Autodesk Fusion 360 part; units mm, degrees
(part 3 of 3)
  measures "d247" diameter of A8
  measures "d248" diameter of A9
  measures "d249" diameter of A10
  measures "d250" diameter of A11
  measures "d251" diameter of A12
  measures "d252" diameter of A13
  measures "d253" diameter of A14
  measures "d254" diameter of A15
  measures "d255" diameter of A16
  measures "d256" diameter of A17
  measures "d257" diameter of A18
  measures "d258" diameter of A19
  measures "d259" diameter of A20
  measures "d260" diameter of A21
  measures "d261" diameter of A22
  measures "d262" diameter of A23
  measures "d263" diameter of A24
  measures "d281" distance of P2 L243.end
  measures "d282" distance of L243.end L244.end
  measures "d283" diameter of A25
  measures "d284" distance of L250.start L249.end
  measures "d285" distance of L250.end L250.start
  measures "d286" diameter of A26
  measures "d287" distance of L255.end L256.end
  measures "d288" distance of L255.start L255.end
  measures "d289" diameter of A30
  measures "d290" diameter of A27
  measures "d291" diameter of A28
  measures "d292" diameter of A29
  measures "d293" distance of L258 L262
  measures "d294" distance of L255 L261
  measures "d295" distance of L276.end L277.end
  measures "d296" distance of L275.end L276.end
  measures "d297" distance of L272.end L273.end
  measures "d298" distance of L271.end L272.end
  measures "d299" distance of L267.start L269.end
extrude "Extruir15" add sketch "Boceto15" along normal blind 4 contours L260 L261 L267 L269 L270 | L259 L260 L271 L272 L273 L274 | L261 L262 L263 L264 L265 L266 | L259 L262 L275 L276 L277 L278 | L151 L152 L153 L154 L157 L158 | L156 L157 L159 L160 L161 L162 | L155 L158 L163 L164 L165 L166 | L155 L156 L167 L168 L169 L170 | L171 L172 L173 L174 | L175 L176 L177 L178 | L179 L180 L181 L182 | L183 L184 L185 L186 | L187 L188 L189 L190 | L191 L192 L193 L194 | L195 L196 L197 L198 | L199 L200 L201 L202 | L203 L204 L205 L206 | L207 L208 L209 L210 | L211 L212 L213 L214 | L215 L216 L217 L218 | L227 L228 L229 L230 | L231 L232 L233 L234 | L235 L236 L237 L238 | L239 L240 L241 L242 | L243 L244 L245 L246 | L249 L250 L252 L254
sketch "Boceto17" plane through (0, 0, 5) normal (0, 0, 1) x (-1, 0, 0)
  circle A0 centre (12, -97) radius 1.5
  circle A1 centre (-162, -97) radius 1.5
  circle A2 centre (12, -3) radius 1.5
  circle A3 centre (-162, -42) radius 1.5
  circle A4 centre (8.65, -85.637) radius 1.6
  circle A5 centre (8.65, -71.337) radius 1.6
  circle A6 centre (-97.75, -72.95) radius 1
  circle A7 centre (-145.75, -75.7793) radius 0.75
  circle A8 centre (-156.15, -6.35) radius 1
  circle A9 centre (-65.25, -19.25) radius 1.5
  circle A10 centre (-24.75, -19.25) radius 1.5
  circle A11 centre (-57.75, -19.25) radius 1.5
  circle A12 centre (-134.75, -64.25) radius 1.5
  circle A13 centre (-155.65, -50.85) radius 1
  circle A14 centre (-104.75, -91.2793) radius 0.75
  circle A15 centre (-77.75, -72.95) radius 1
  circle A16 centre (-16.9746, -57.735) radius 1.4
  circle A17 centre (4.6254, -28.735) radius 1.4
  circle A18 centre (4.6254, -57.735) radius 1.25
  circle A19 centre (-97.75, -89.75) radius 1
  circle A20 centre (-145.75, -91.2793) radius 0.75
  circle A21 centre (-141.85, -6.35) radius 1
  circle A22 centre (-65.25, -64.25) radius 1.5
  circle A23 centre (-24.75, -64.25) radius 1.5
  circle A24 centre (-57.75, -64.25) radius 1.5
  circle A25 centre (-134.75, -19.25) radius 1.5
  circle A26 centre (-155.75, -65.15) radius 1
  circle A27 centre (-104.75, -75.7793) radius 0.75
  circle A28 centre (-77.75, -89.75) radius 1
  circle A29 centre (-16.9746, -28.735) radius 1.4
  line L0 (-165, 0) -> (-165, -77.5293)
extrude "Extruir24" cut sketch "Boceto17" against normal blind 90 contours A0 | A1 | A2 | A3
sketch "Boceto16" plane through (0, 0, 5) normal (0, 0, 1) x (-1, 0, 0)
  line L0 (-157.5, -63) -> (-159, -63)
  line L1 (-165, -77.5293) -> (-147, -77.5293)
  line L2 (-147, -77.5293) -> (-147, -77.0293)
  line L3 (-144.5, -74.5293) -> (-106, -74.5293)
  line L4 (-103.5, -77.0293) -> (-103.5, -90.0293)
  line L5 (-106, -92.5293) -> (-144.5, -92.5293)
  line L6 (-147, -89.5293) -> (-165, -89.5293)
  line L7 (-165, -89.5293) -> (-165, -100)
  line L8 (-165, -100) -> (15, -100)
  line L9 (15, -100) -> (15, 0)
  line L10 (10.5, -83.487) -> (10.5, -83.787)
  line L11 (6.8, -87.487) -> (-7.5, -87.487)
  line L12 (-7.5, -87.487) -> (-7.5, -69.487)
  line L13 (-7.5, -69.487) -> (6.8, -69.487)
  line L14 (10.5, -73.487) -> (12, -73.487)
  line L15 (15, 0) -> (-165, 0)
  line L16 (-144, -3) -> (-144, -4.5)
  line L17 (-140, -8.2) -> (-140, -22.5)
  line L18 (-140, -22.5) -> (-158, -22.5)
  line L19 (-158, -22.5) -> (-158, -8.2)
  line L20 (-154, -4.5) -> (-154, -3)
  line L21 (-159, -53) -> (-157.5, -53)
  line L22 (-157.5, -53) -> (-157.5, -52.7)
  line L23 (-153.8, -49) -> (-139.5, -49)
  line L24 (-139.5, -49) -> (-139.5, -67)
  line L25 (-139.5, -67) -> (-153.8, -67)
  line L26 (-60.5, -61.5) -> (-60.5, -22)
  line L27 (-55, -16.5) -> (-27.5, -16.5)
  line L28 (-22, -22) -> (-22, -61.5)
  line L29 (-27.5, -67) -> (-55, -67)
  line L30 (-100.5, -87) -> (-100.5, -75.7)
  line L31 (-95, -70.2) -> (-80.5, -70.2)
  line L32 (-75, -75.7) -> (-75, -87)
  line L33 (-80.5, -92.5) -> (-95, -92.5)
  line L34 (-72.5, -92.5) -> (-72.5, -69)
  line L35 (-72.5, -69) -> (-22, -69)
  line L36 (-22, -69) -> (-22, -92.5)
  line L37 (-22, -92.5) -> (-72.5, -92.5)
  line L38 (-19.3746, -53.685) -> (-19.3746, -32.785)
  line L39 (-13.3746, -24.785) -> (1.0254, -24.785)
  line L40 (7.0254, -32.785) -> (7.0254, -53.685)
  line L41 (1.0254, -61.685) -> (-13.3746, -61.685)
  line L42 (-137.5, -61.5) -> (-137.5, -22)
  line L43 (-132, -16.5) -> (-68, -16.5)
  line L44 (-62.5, -22) -> (-62.5, -61.5)
  line L45 (-68, -67) -> (-132, -67)
  line L46 (-132.793, -73.7793) -> (-132.793, -67.7793)
  line L47 (-132.793, -67.7793) -> (-112.793, -67.7793)
  line L48 (-112.793, -67.7793) -> (-112.793, -73.7793)
  line L49 (-112.793, -73.7793) -> (-132.793, -73.7793)
  line L50 (163.4623, -50) -> (102.1469, -50)
  line L51 (102.1469, -50) -> (102.1469, -3.728)
  line L52 (102.1469, -3.728) -> (163.4623, -3.728)
  line L53 (163.4623, -3.728) -> (163.4623, -50)
  circle A0 centre (158.4623, -45) radius 1.5
  line L54 (163.4623, -40) -> (158.4623, -40)
  line L55 (153.4623, -50) -> (153.4623, -45)
  arc A1 (158.4623, -40) -> (153.4623, -45) centre (158.4623, -45) ccw
  line L56 (9, 0) -> (9, -3)
  line L57 (12, -6) -> (12, -6)
  arc A2 (15, -3.0005) -> (15, -2.9995) centre (12, -3) ccw
  arc A3 (9, -3) -> (12, -6) centre (12, -3) ccw
  line L58 (-162, -45) -> (-165, -45)
  line L59 (-165, -39) -> (-162, -39)
  arc A4 (-162, -45) -> (-162, -39) centre (-162, -42) ccw
  line L60 (-154.4341, -89.5293) -> (-154.4341, -77.5293)
  line L61 (-162, -94) -> (-160, -94)
  line L62 (-159, -100) -> (-159, -97)
  arc A5 (-159, -97) -> (-162, -94) centre (-162, -97) ccw
  line L63 (15, -94) -> (12, -94)
  line L64 (9, -100) -> (9, -97)
  arc A6 (12, -94) -> (9, -97) centre (12, -97) ccw
  line L65 (12, -97) -> (-162, -97)
  line L66 (-162, -97) -> (-162, -3)
  line L67 (-162, -3) -> (12, -3)
  line L68 (12, -3) -> (12, -97)
  line L69 (12, -73.487) -> (12, -83.487)
  line L70 (12, -83.487) -> (10.5, -83.487)
  line L71 (-159, -63) -> (-159, -53)
  line L72 (-154.3, -4.5) -> (-154, -4.5)
  line L73 (-154, -3) -> (-144, -3)
  line L74 (-165, -89.5293) -> (-165, -77.5293)
  circle A7 centre (12, -97) radius 1.5
  circle A8 centre (-162, -97) radius 1.5
  circle A9 centre (12, -3) radius 1.5
  circle A10 centre (-162, -42) radius 1.5
  circle A11 centre (8.65, -85.637) radius 1.6
  circle A12 centre (8.65, -71.337) radius 1.6
  circle A13 centre (-97.75, -72.95) radius 1
  circle A14 centre (-145.75, -75.7793) radius 0.75
  circle A15 centre (-156.15, -6.35) radius 1
  circle A16 centre (-65.25, -19.25) radius 1.5
  circle A17 centre (-24.75, -19.25) radius 1.5
  circle A18 centre (-57.75, -19.25) radius 1.5
  circle A19 centre (-134.75, -64.25) radius 1.5
  circle A20 centre (-155.65, -50.85) radius 1
  circle A21 centre (-104.75, -91.2793) radius 0.75
  circle A22 centre (-77.75, -72.95) radius 1
  circle A23 centre (-16.9746, -57.735) radius 1.4
  circle A24 centre (4.6254, -28.735) radius 1.4
  circle A25 centre (4.6254, -57.735) radius 1.25
  circle A26 centre (-97.75, -89.75) radius 1
  circle A27 centre (-145.75, -91.2793) radius 0.75
  circle A28 centre (-141.85, -6.35) radius 1
  circle A29 centre (-65.25, -64.25) radius 1.5
  circle A30 centre (-24.75, -64.25) radius 1.5
  circle A31 centre (-57.75, -64.25) radius 1.5
  circle A32 centre (-134.75, -19.25) radius 1.5
  circle A33 centre (-155.75, -65.15) radius 1
  circle A34 centre (-104.75, -75.7793) radius 0.75
  circle A35 centre (-77.75, -89.75) radius 1
  circle A36 centre (-16.9746, -28.735) radius 1.4
  line L75 (-147, -77.0293) -> (-144.5, -77.0293)
  line L76 (-144.5, -77.0293) -> (-144.5, -74.5293)
  line L77 (-106, -74.5293) -> (-106, -77.0293)
  line L78 (-106, -77.0293) -> (-103.5, -77.0293)
  line L79 (-103.5, -90.0293) -> (-106, -90.0293)
  line L80 (-106, -90.0293) -> (-106, -92.5293)
  line L81 (-144.5, -92.5293) -> (-144.5, -90.0293)
  line L82 (-144.5, -90.0293) -> (-147, -90.0293)
  line L83 (-147, -90.0293) -> (-147, -89.5293)
  line L84 (-165, 0) -> (-165, -77.5293)
  line L85 (10.5, -83.787) -> (6.8, -83.787)
  line L86 (6.8, -83.787) -> (6.8, -87.487)
  line L87 (6.8, -69.487) -> (6.8, -73.187)
  line L88 (6.8, -73.187) -> (10.5, -73.187)
  line L89 (10.5, -73.187) -> (10.5, -73.487)
  line L90 (-137.5, -22) -> (-132, -22)
  line L91 (-132, -22) -> (-132, -16.5)
  line L92 (-68, -16.5) -> (-68, -22)
  line L93 (-68, -22) -> (-62.5, -22)
  line L94 (-62.5, -61.5) -> (-68, -61.5)
  line L95 (-68, -61.5) -> (-68, -67)
  line L96 (-132, -67) -> (-132, -61.5)
  line L97 (-132, -61.5) -> (-137.5, -61.5)
  line L98 (-19.3746, -32.785) -> (-13.3746, -32.785)
  line L99 (-13.3746, -32.785) -> (-13.3746, -24.785)
  line L100 (1.0254, -24.785) -> (1.0254, -32.785)
  line L101 (1.0254, -32.785) -> (7.0254, -32.785)
  line L102 (7.0254, -53.685) -> (1.0254, -53.685)
  line L103 (1.0254, -53.685) -> (1.0254, -61.685)
  line L104 (-13.3746, -61.685) -> (-13.3746, -53.685)
  line L105 (-13.3746, -53.685) -> (-19.3746, -53.685)
  line L106 (-144, -4.5) -> (-143.7, -4.5)
  line L107 (-143.7, -4.5) -> (-143.7, -8.2)
  line L108 (-143.7, -8.2) -> (-140, -8.2)
  line L109 (-158, -8.2) -> (-154.3, -8.2)
  line L110 (-154.3, -8.2) -> (-154.3, -4.5)
  line L111 (-100.5, -75.7) -> (-95, -75.7)
  line L112 (-95, -75.7) -> (-95, -70.2)
  line L113 (-80.5, -70.2) -> (-80.5, -75.7)
  line L114 (-80.5, -75.7) -> (-75, -75.7)
  line L115 (-75, -87) -> (-80.5, -87)
  line L116 (-80.5, -87) -> (-80.5, -92.5)
  line L117 (-95, -92.5) -> (-95, -87)
  line L118 (-95, -87) -> (-100.5, -87)
  line L119 (-60.5, -22) -> (-55, -22)
  line L120 (-55, -22) -> (-55, -16.5)
  line L121 (-27.5, -16.5) -> (-27.5, -22)
  line L122 (-27.5, -22) -> (-22, -22)
  line L123 (-22, -61.5) -> (-27.5, -61.5)
  line L124 (-27.5, -61.5) -> (-27.5, -67)
  line L125 (-55, -67) -> (-55, -61.5)
  line L126 (-55, -61.5) -> (-60.5, -61.5)
  line L127 (-157.5, -52.7) -> (-153.8, -52.7)
  line L128 (-153.8, -52.7) -> (-153.8, -49)
  line L129 (-153.8, -67) -> (-153.8, -63.3)
  line L130 (-153.8, -63.3) -> (-157.5, -63.3)
  line L131 (-157.5, -63.3) -> (-157.5, -63)
  dimension "d302" = 5
  dimension "d303" = 5
  dimension "d304" = 10
  dimension "d305" = 3
  dimension "d306" = 3
  dimension "d307" = 3
  constraint horizontal L50
  constraint vertical L51
  constraint horizontal L52
  constraint vertical L53
  constraint concentric A0 A1
  constraint coincident L53 L54.start
  constraint perpendicular L53 L54
  constraint coincident L50 L55.start
  constraint perpendicular L50 L55
  constraint tangent L55 A1
  constraint tangent L54 A1
  constraint tangent L15 A2
  constraint coincident L15 L56.start
  constraint perpendicular L15 L56
  constraint tangent L57 A2
  constraint tangent L56 A2
  constraint coincident L56.end A2
  constraint concentric A2 A3
  constraint tangent L59 A4
  constraint tangent L58 A4
  constraint coincident L6 L60.start
  constraint coincident L1 L60.end
  constraint perpendicular L1 L60
  constraint tangent L8 A5
  constraint coincident L61.start A5
  constraint horizontal L61
  constraint coincident L8 L62.start
  constraint perpendicular L8 L62
  constraint tangent L62 A5
  constraint coincident L61 A5.end
  constraint tangent L9 A6
  constraint coincident L9 L63.start
  constraint perpendicular L9 L63
  constraint coincident L8 L64.start
  constraint perpendicular L8 L64
  constraint tangent L64 A6
  constraint tangent L63 A6
  constraint horizontal L65
  constraint vertical L66
  constraint horizontal L67
  constraint vertical L68
  constraint coincident L68 L57.start
  measures "d302" distance of L50 A0.centre
  measures "d303" distance of L53 A0.centre
  measures "d304" diameter of A1
  measures "d305" diameter of A0
  measures "d306" distance of L15 L67
  measures "d307" distance of L8 L65
extrude "Extruir23" add sketch "Boceto16" along normal blind 50 contours L1 L6 L66 L74 | L1 L58 L66 L84 | L6 L7 L8 L62 L65 L66 A8 | A4 L66 A10 | L58 L59 L66 A10 L84 | A5 L65 L66 A8 | L15 L56 L59 L66 L67 L73 L84 | L8 L62 L64 L65 | L8 L9 L63 L64 L65 L68 A7 | A6 L65 L68 A7 | L15 L56 A2 | L9 A2 L63 L68 L69 | L9 L15 A2 | A2 L67 L68 A9 | A2 A3 L67 L68 A9
extrude "Extruir25" add 1 faces at (163, 85.5293, 5) along direction (0, 0, -1) blind 4
sketch "Boceto18" plane through (165, 0, 0) normal (1, 0, 0) x (0, 1, 0)
  line L0 (100, 0) -> (100, 55)
  line L1 (100, 55) -> (0, 55)
  line L2 (0, 55) -> (0, 0)
  line L3 (0, 0) -> (100, 0)
  line L4 (49, 1) -> (52.7, 1) construction
  line L5 (52.7, 1) -> (53, 1) construction
  line L6 (53, 1) -> (63, 1) construction
  line L7 (63, 1) -> (63.3, 1) construction
  line L8 (63.3, 1) -> (67, 1) construction
  line L9 (67, 1) -> (49, 1) construction
  line L10 (53.45, 5) -> (62.55, 5) construction
  line L11 (62.55, 5) -> (62.55, 2) construction
  line L12 (62.55, 2) -> (53.45, 2) construction
  line L13 (53.45, 2) -> (53.45, 5) construction
  line L14 (58, 1) -> (58, 2) construction
  line L15 (54.95, 2) -> (61.05, 2) construction
  arc A0 (61.05, 2) -> (61.05, 5) centre (61.05, 3.5) ccw construction
  line L16 (61.05, 5) -> (54.95, 5) construction
  arc A1 (54.95, 5) -> (54.95, 2) centre (54.95, 3.5) ccw construction
  line L17 (53.45, 3.5) -> (62.55, 3.5) construction
  arc A2 (61.05, -1) -> (61.05, 8) centre (61.05, 3.5) ccw
  line L18 (61.05, 8) -> (54.95, 8)
  arc A3 (54.95, 8) -> (54.95, -1) centre (54.95, 3.5) ccw
  line L19 (54.95, -1) -> (61.05, -1)
  line L20 (50.45, 3.5) -> (50.45, 0)
  line L21 (65.55, 3.5) -> (65.55, 0)
  point P0 (49, 1)
  dimension "d322" = 1
  dimension "d323" = 3
  dimension "d324" = 9.1
  dimension "d325" = 3
  constraint horizontal L10
  constraint vertical L11
  constraint horizontal L12
  constraint vertical L13
  constraint midpoint L6 L14.start
  constraint midpoint L12 L14.end
  constraint vertical L14
  constraint tangent L15 A0
  constraint tangent A0 L16
  constraint parallel L15 L16
  constraint tangent L16 A1
  constraint tangent L15 A1
  constraint midpoint A1 L17.start
  constraint midpoint A0 L17.end
  constraint midpoint L11 L17.end
  constraint perpendicular L11 L17
  constraint midpoint L13 L17.start
  constraint midpoint A3 L20.start
  constraint coincident L3 L20.end
  constraint tangent A3 L20
  constraint perpendicular L3 L20
  constraint midpoint A2 L21.start
  constraint coincident L3 L21.end
  constraint tangent A2 L21
  constraint perpendicular L3 L21
  measures "d322" distance of L9 L12
  measures "d323" distance of L10.end L11.end
  measures "d324" distance of L10.start L10.end
extrude "Extruir26" cut sketch "Boceto18" against normal blind 6 contours L3 A2 L21 | L3 A2 L18 A3 | L3 A3 L20
sketch "Boceto19" plane through (0, 0, 0) normal (0, -1, 0) x (1, 0, 0)
  line L0 (-15, 0) -> (165, 0)
  line L1 (165, 0) -> (165, 55)
  line L2 (165, 55) -> (-15, 55)
  line L3 (-15, 55) -> (-15, 0)
  line L4 (152.0391, 4.1783) -> (145.9609, 4.1783) construction
  line L5 (140.8268, 0.1675) -> (144.0809, 1) construction
  line L6 (144.45, 1.1675) -> (144.45, 4.1675) construction
  line L7 (145.9609, 1.1566) -> (152.0391, 1.1566) construction
  line L8 (153.9217, 1) -> (157.1517, 0.1675) construction
  line L9 (144.45, 4.1675) -> (153.55, 4.1675) construction
  line L10 (152.0391, 7.1783) -> (145.9608, 7.1783)
  arc A0 (145.9609, 4.1783) -> (145.9609, 1.1566) centre (145.9609, 2.6675) ccw construction
  line L11 (141.45, 2.6675) -> (141.45, -2.9323)
  line L12 (148.9999, 1) -> (153.9217, 1) construction
  line L13 (144.0809, 1) -> (149.0001, 1) construction
  line L14 (144.45, 2.6675) -> (153.55, 2.6675) construction
  arc A1 (152.0392, -1.8434) -> (152.0391, 7.1783) centre (152.0391, 2.6675) ccw
  line L15 (149.0001, 1) -> (148.9999, 1) construction
  line L16 (153.55, 4.1675) -> (153.55, 1.1675) construction
  line L17 (157.1517, 0.1675) -> (140.8268, 0.1675) construction
  arc A2 (152.0391, 1.1566) -> (152.0391, 4.1783) centre (152.0391, 2.6675) ccw construction
  arc A3 (145.9608, 7.1783) -> (145.9608, -1.8434) centre (145.9609, 2.6675) ccw
  line L18 (153.55, 1.1675) -> (144.45, 1.1675) construction
  line L19 (156.55, 2.6675) -> (156.5501, -3.4458)
  line L20 (145.9608, -1.8434) -> (152.0392, -1.8434)
  line L21 (149, 1) -> (149, 1.1675) construction
  line L22 (154.3, 1) -> (158, 1) construction
  line L23 (158, 1) -> (140, 1) construction
  line L24 (140, 1) -> (143.7, 1) construction
  line L25 (143.7, 1) -> (144, 1) construction
  line L26 (144, 1) -> (154, 1) construction
  line L27 (154, 1) -> (154.3, 1) construction
  point P0 (61.5347, -18.624)
  point P1 (149, 1)
  dimension "d328" = 3
  dimension "d329" = 1
  dimension "d330" = 3
  dimension "d331" = 9.1
  constraint horizontal L9
  constraint vertical L16
  constraint horizontal L18
  constraint vertical L6
  constraint midpoint P1 L15
  constraint midpoint L21.end L18
  constraint vertical L21
  constraint tangent L7 A2
  constraint tangent L4 A2
  constraint parallel L4 L7
  constraint tangent L4 A0
  constraint tangent L7 A0
  constraint midpoint L14.start A0
  constraint midpoint L14.end A2
  constraint midpoint L14.end L16
  constraint perpendicular L14 L16
  constraint midpoint L14.start L6
  constraint midpoint L11.start A3
  constraint tangent L11 A3
  constraint midpoint L19.start A1
  constraint tangent A1 L19
  constraint midpoint L26 P1
  constraint coincident P1 L21.start
  measures "d329" distance of L17 L18
  measures "d330" distance of L16.end L9.end
  measures "d331" distance of L6.end L9.end
extrude "Extruir27" cut sketch "Boceto19" against normal blind 3 contours L0 L11 A3 | L0 L10 A1 A3 | L0 A1 L19
sketch "Boceto20" plane through (-15, 0, 0) normal (-1, 0, 0) x (0, -1, 0)
  line L0 (-100, 0) -> (0, 0)
  line L1 (0, 0) -> (0, 55)
  line L2 (0, 55) -> (-2.9995, 55)
  line L3 (-2.9995, 55) -> (-2.9995, 5)
  line L4 (-2.9995, 5) -> (-3.0005, 5)
  line L5 (-3.0005, 55) -> (-100, 55)
  line L6 (-100, 55) -> (-100, 0)
  line L7 (-75.437, 5) -> (-81.537, 5) construction
  line L8 (-87.487, 1) -> (-83.787, 1) construction
  line L9 (-83.037, 2) -> (-83.037, 5) construction
  line L10 (-81.537, 2) -> (-75.437, 2) construction
  line L11 (-73.187, 1) -> (-69.487, 1) construction
  line L12 (-83.037, 5) -> (-73.937, 5) construction
  line L13 (-75.437, 8) -> (-81.537, 8)
  arc A0 (-81.537, 5) -> (-81.537, 2) centre (-81.537, 3.5) ccw construction
  line L14 (-86.037, 3.5) -> (-86.037, 0)
  line L15 (-73.487, 1) -> (-73.187, 1) construction
  line L16 (-83.787, 1) -> (-83.487, 1) construction
  line L17 (-83.037, 3.5) -> (-73.937, 3.5) construction
  arc A1 (-75.437, -1) -> (-75.437, 8) centre (-75.437, 3.5) ccw
  line L18 (-83.487, 1) -> (-73.487, 1) construction
  line L19 (-73.937, 5) -> (-73.937, 2) construction
  line L20 (-69.487, 1) -> (-87.487, 1) construction
  arc A2 (-75.437, 2) -> (-75.437, 5) centre (-75.437, 3.5) ccw construction
  arc A3 (-81.537, 8) -> (-81.537, -1) centre (-81.537, 3.5) ccw
  line L21 (-73.937, 2) -> (-83.037, 2) construction
  line L22 (-70.937, 3.5) -> (-70.937, 0)
  line L23 (-81.537, -1) -> (-75.437, -1)
  line L24 (-78.487, 1) -> (-78.487, 2) construction
  line L25 (-87.487, 1) -> (-83.787, 1) construction
  line L26 (-83.787, 1) -> (-83.487, 1) construction
  line L27 (-83.487, 1) -> (-73.487, 1) construction
  line L28 (-73.487, 1) -> (-73.187, 1) construction
  line L29 (-73.187, 1) -> (-69.487, 1) construction
  line L30 (-69.487, 1) -> (-87.487, 1) construction
  line L31 (-3.0005, 5) -> (-3.0005, 55)
  point P0 (49, 1)
  point P1 (-78.487, 1)
  dimension "d334" = 3
  dimension "d335" = 1
  dimension "d336" = 3
  dimension "d337" = 9.1
  constraint horizontal L12
  constraint vertical L19
  constraint horizontal L21
  constraint vertical L9
  constraint midpoint P1 L18
  constraint midpoint L24.end L21
  constraint vertical L24
  constraint tangent L10 A2
  constraint tangent L7 A2
  constraint parallel L7 L10
  constraint tangent L7 A0
  constraint tangent L10 A0
  constraint midpoint L17.start A0
  constraint midpoint L17.end A2
  constraint midpoint L17.end L19
  constraint perpendicular L17 L19
  constraint midpoint L17.start L9
  constraint midpoint L14.start A3
  constraint tangent L14 A3
  constraint midpoint L22.start A1
  constraint tangent A1 L22
  constraint midpoint L27 P1
  constraint coincident P1 L24.start
  measures "d335" distance of L20 L21
  measures "d336" distance of L19.end L12.end
  measures "d337" distance of L9.end L12.end
extrude "Extruir28" cut sketch "Boceto20" against normal blind 3 contours L0 L14 A3 | L0 L13 A1 A3 | L0 A1 L22
sketch "Boceto21" plane through (0, 0, 0) normal (0, -1, 0) x (1, 0, 0)
  line L0 (156.55, 2.6675) -> (156.5501, 0)
  line L1 (156.5501, 0) -> (165, 0)
  line L2 (165, 0) -> (165, 55)
  line L3 (165, 55) -> (-15, 55)
  line L4 (-15, 55) -> (-15, 0)
  line L5 (-15, 0) -> (141.45, 0)
  line L6 (141.45, 0) -> (141.45, 2.6675)
  arc A0 (145.9608, 7.1783) -> (141.45, 2.6675) centre (145.9609, 2.6675) ccw
  line L7 (145.9608, 7.1783) -> (152.0391, 7.1783)
  arc A1 (156.55, 2.6675) -> (152.0391, 7.1783) centre (152.0391, 2.6675) ccw
  circle A2 centre (70.8934, 40) radius 9.75
  circle A3 centre (129.1066, 40) radius 6.45
  line L8 (62.5, 5) -> (137.5, 5) construction
  line L9 (100, 5) -> (100, 40) construction
  line L10 (70.8934, 40) -> (129.1066, 40) construction
  point P0 (62.5, 5)
  point P1 (137.5, 5)
  dimension "d340" = 19.5
  dimension "d341" = 12.9
  dimension "d342" = 35
  constraint coincident P0 L8.start
  constraint coincident P1 L8.end
  constraint midpoint L8 L9.start
  constraint perpendicular L8 L9
  constraint coincident A2.centre L10.start
  constraint coincident A3.centre L10.end
  constraint horizontal L10
  constraint midpoint L9.end L10
  measures "d340" diameter of A2
  measures "d341" diameter of A3
  measures "d342" distance of L9.start L9.end
extrude "Extruir29" cut sketch "Boceto21" against normal blind 3 contours A2 | A3
sketch "Boceto22" plane through (0, 100, 0) normal (0, 1, 0) x (-1, 0, 0)
  line L0 (-165, 0) -> (15, 0)
  line L1 (15, 0) -> (15, 55)
  line L2 (15, 55) -> (-165, 55)
  line L3 (-165, 55) -> (-165, 0)
  line L4 (-72.5, 5) -> (-72.5, 6)
  line L5 (-72.5, 6) -> (-72.5, 33) construction
  line L6 (-22, 5) -> (-22, 34.9) construction
  circle A0 centre (-22, 37.1) radius 1.8
  circle A1 centre (-22, 17.9) radius 1.8
  line L7 (-22, 37.1) -> (-22, 17.9) construction
  line L8 (-22, 27.5) -> (15, 27.5) construction
  line L9 (-22, 27.5) -> (-79, 27.5) construction
  circle A2 centre (-72.5, 27.5) radius 2
  point P0 (-72.5, 5)
  point P1 (-22, 5)
  dimension "d345" = 3.6
  dimension "d346" = 3.6
  dimension "d347" = 19.2
  dimension "d350" = 4
  constraint coincident P0 L4.start
  constraint perpendicular L0 L4
  constraint perpendicular L0 L5
  constraint coincident P1 L6.start
  constraint perpendicular L0 L6
  constraint coincident L6 A0.centre
  constraint coincident L6 A1.centre
  constraint coincident A0.centre L7.start
  constraint coincident A1.centre L7.end
  constraint midpoint L7 L8.start
  constraint midpoint L1 L8.end
  constraint horizontal L8
  constraint perpendicular L5 L9
  constraint coincident L9 A2.centre
  constraint coincident L5 A2.centre
  measures "d345" diameter of A0
  measures "d346" diameter of A1
  measures "d347" distance of A0.centre A1.centre
  measures "d350" diameter of A2
extrude "Extruir30" cut sketch "Boceto22" against normal blind 3 contours A0 | A1 | A2
fillet "Empalme1" radius 2 4 edges at (165, 100, 27.5) (-15, 100, 27.5) (-15, 0, 27.5) (165, 0, 27.5)
sketch "Boceto23" plane through (0, 0, 5) normal (0, 0, 1) x (-1, 0, 0)
  circle A0 centre (-16.9746, -28.735) radius 1.4
  circle A1 centre (-77.75, -89.75) radius 1
  circle A2 centre (-104.75, -75.7793) radius 0.75
  circle A3 centre (-155.75, -65.15) radius 1
  circle A4 centre (-134.75, -19.25) radius 1.5
  circle A5 centre (-57.75, -64.25) radius 1.5
  circle A6 centre (-24.75, -64.25) radius 1.5
  circle A7 centre (-65.25, -64.25) radius 1.5
  circle A8 centre (-141.85, -6.35) radius 1
  circle A9 centre (-145.75, -91.2793) radius 0.75
  circle A10 centre (-97.75, -89.75) radius 1
  circle A11 centre (4.6254, -57.735) radius 1.25
  circle A12 centre (4.6254, -28.735) radius 1.4
  circle A13 centre (-16.9746, -57.735) radius 1.4
  circle A14 centre (-77.75, -72.95) radius 1
  circle A15 centre (-104.75, -91.2793) radius 0.75
  circle A16 centre (-155.65, -50.85) radius 1
  circle A17 centre (-134.75, -64.25) radius 1.5
  circle A18 centre (-57.75, -19.25) radius 1.5
  circle A19 centre (-24.75, -19.25) radius 1.5
  circle A20 centre (-65.25, -19.25) radius 1.5
  circle A21 centre (-156.15, -6.35) radius 1
  circle A22 centre (-145.75, -75.7793) radius 0.75
  circle A23 centre (-97.75, -72.95) radius 1
  circle A24 centre (8.65, -71.337) radius 1.6
  circle A25 centre (8.65, -85.637) radius 1.6
extrude "Extruir31" cut sketch "Boceto23" against normal blind 210
equation "d268 = ( 1.5 / 2 ) * 1 mm"
equation "d287 = 26 mm + 3 mm"
equation "d288 = 18.6 mm + 3 mm"
equation "d293 = ( 26.4 - 21.6 ) / 2 * 1 mm"
equation "d294 = ( 7.9 / 2 ) * 1 mm"
equation "d340 = 19.2 mm + 0.3 mm"
equation "d341 = 12.6 mm + 0.3 mm"
equation "d347 = 15.6 mm + 3.6 mm"
